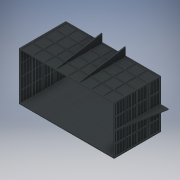
# Autodesk Inventor part: pool cut
Saved by Autodesk Inventor 2019 (Build 230136000, 136)
## iProperties
Created: 2021-05-11
Part Number: pool cut
Material: Stainless Steel, Austenitic
Document SubType Name: Modeling
Designer: jamieson-bl
Density: 8 g/cm^3
Appearance: Semi-Polished
Author: jamieson-bl
Autodesk Inventor part; units mm, degrees
ref_plane "YZ Plane" through (0, 0, 0) normal (1, 0, 0) x (0, 1, 0)
ref_plane "XZ Plane" through (0, 0, 0) normal (0, 1, 0) x (-1, 0, 0)
ref_plane "XY Plane" through (0, 0, 0) normal (0, 0, 1) x (1, 0, 0)
sketch "Sketch1" plane through (0, 0, 0) normal (0, 0, 1) x (1, 0, 0)
  line L0 (1524, -762) -> (-1524, -762)
  line L1 (-1524, -762) -> (-1524, 762)
  line L2 (-1524, 762) -> (1524, 762)
  line L3 (1524, 762) -> (1524, -762)
  line L4 (1524, -762) -> (-1524, 762) construction
  line L5 (-1524, -762) -> (1524, 762) construction
  point P0 (0, 0)
  dimension "d0" = 3048
  dimension "d1" = 1524
  constraints: 12 end point, 2 midpoint, 2 parallel, 1 horizontal, 1 perpendicular
  measures "d0" distance of L1.end L2.end
  measures "d1" distance of L0.end L1.end
extrude "Extrusion1" add sketch "Sketch1" along normal blind 1524
sketch "Sketch2" plane through (0, 0, 1524) normal (0, 0, 1) x (1, 0, 0)
  line L0 (1521.333, -759.333) -> (-1521.333, -759.333)
  line L1 (-1521.333, -759.333) -> (-1521.333, 759.333)
  line L2 (-1521.333, 759.333) -> (1521.333, 759.333)
  line L3 (1521.333, 759.333) -> (1521.333, -759.333)
  line L4 (1521.333, -759.333) -> (-1521.333, 759.333) construction
  line L5 (-1521.333, -759.333) -> (1521.333, 759.333) construction
  point P0 (0, 0)
  dimension "d4" = 3042.666
  dimension "d5" = 1518.666
  constraints: 12 end point, 2 midpoint, 2 parallel, 1 horizontal, 1 perpendicular
  measures "d4" distance of L1.end L2.end
  measures "d5" distance of L0.end L1.end
extrude "Extrusion2" cut sketch "Sketch2" against normal blind 1521.333
sketch "Sketch12" plane through (-1524, 762, 0) normal (0, 1, 0) x (1, 0, 0)
  line L0 (-182.8526, -1524) -> (4734.6574, -1524)
  line L1 (0, -1524) -> (3048, -1524) projected
  line L2 (4734.6574, -1524) -> (4734.6574, -1424)
  line L3 (4734.6574, -1424) -> (-182.8526, -1424)
  line L4 (-182.8526, -1424) -> (-182.8526, -1324)
  line L5 (-182.8526, -1324) -> (4734.6574, -1324)
  line L6 (4734.6574, -1324) -> (4734.6574, -1224)
  line L7 (4734.6574, -1224) -> (-182.8526, -1224)
  line L8 (-182.8526, -1224) -> (-182.8526, -1124)
  line L9 (-182.8526, -1124) -> (4734.6574, -1124)
  line L10 (4734.6574, -1124) -> (4734.6574, -1024)
  line L11 (4734.6574, -1024) -> (-182.8526, -1024)
  line L12 (-182.8526, -1024) -> (-182.8526, -924)
  line L13 (-182.8526, -924) -> (4734.6574, -924)
  line L14 (4734.6574, -924) -> (4734.6574, -824)
  line L15 (4734.6574, -824) -> (-182.8526, -824)
  line L16 (-182.8526, -824) -> (-182.8526, -724)
  line L17 (-182.8526, -724) -> (4734.6574, -724)
  line L18 (4734.6574, -724) -> (4734.6574, -624)
  line L19 (4734.6574, -624) -> (-182.8526, -624)
  line L20 (-182.8526, -624) -> (-182.8526, -524)
  line L21 (-182.8526, -524) -> (4734.6574, -524)
  line L22 (4734.6574, -524) -> (4734.6574, -424)
  line L23 (4734.6574, -424) -> (-182.8526, -424)
  line L24 (-182.8526, -424) -> (-182.8526, -324)
  line L25 (-182.8526, -324) -> (4734.6574, -324)
  line L26 (4734.6574, -324) -> (4734.6574, -224)
  line L27 (4734.6574, -224) -> (-182.8526, -224)
  line L28 (-182.8526, -224) -> (-182.8526, -124)
  line L29 (-182.8526, -124) -> (4734.6574, -124)
  point P0 (1524, 0)
  dimension "d46" = 100
  dimension "d47" = 100
  dimension "d48" = 100
  dimension "d49" = 100
  dimension "d50" = 100
  dimension "d51" = 100
  dimension "d52" = 100
  dimension "d53" = 100
  dimension "d54" = 100
  dimension "d55" = 100
  dimension "d56" = 100
  dimension "d57" = 100
  dimension "d58" = 100
  dimension "d59" = 100
  constraints: 58 end point, 25 point on line, 11 perpendicular, 5 parallel, 1 collinear
  measures "d46" distance of L0.end L2.end
  measures "d47" distance of L3.end L4.end
  measures "d48" distance of L5.end L6.end
  measures "d49" distance of L7.end L8.end
  measures "d50" distance of L9.end L10.end
  measures "d51" distance of L11.end L12.end
  measures "d52" distance of L13.end L14.end
  measures "d53" distance of L15.end L16.end
  measures "d54" distance of L17.end L18.end
  measures "d55" distance of L19.end L20.end
  measures "d56" distance of L21.end L22.end
  measures "d57" distance of L23.end L24.end
  measures "d58" distance of L25.end L26.end
  measures "d59" distance of L27.end L28.end
split_face "Split8"
sketch "Sketch15" plane through (0, 0, 0) normal (0, 0, -1) x (-1, 0, 0)
  line L0 (-1524, 762) -> (-1524, -762) projected
  line L1 (-1524, 762) -> (-1524, 758.825)
  line L2 (-1549.4, 758.825) -> (-1549.4, 787.4)
  line L3 (-1549.4, 787.4) -> (-1498.6, 787.4)
  line L4 (-1498.6, 787.4) -> (-1498.6, 762)
  line L5 (1524, 762) -> (-1524, 762) projected
  line L6 (-1498.6, 762) -> (-1524, 762)
  line L7 (-1549.4, 758.825) -> (-1524, 758.825)
  line L8 (1549.4, -758.825) -> (1524, -758.825)
  line L9 (1549.4, -758.825) -> (1549.4, -787.4)
  line L10 (1549.4, -787.4) -> (1498.6, -787.4)
  line L11 (1498.6, -787.4) -> (1498.6, -762)
  line L12 (1498.6, -762) -> (1524, -762)
  line L13 (1524, -762) -> (1524, -758.825)
  line L14 (0, 0) -> (657.5031, 0) construction
  line L15 (-1524, -762) -> (-1524, 762)
  line L16 (-1524, -762) -> (-1524, -758.825)
  line L17 (-1549.4, -758.825) -> (-1549.4, -787.4)
  line L18 (-1549.4, -787.4) -> (-1498.6, -787.4)
  line L19 (-1498.6, -787.4) -> (-1498.6, -762)
  line L20 (1524, -762) -> (-1524, -762)
  line L21 (-1549.4, -758.825) -> (-1524, -758.825)
  line L22 (1549.4, 758.825) -> (1524, 758.825)
  line L23 (1549.4, 758.825) -> (1549.4, 787.4)
  line L24 (1549.4, 787.4) -> (1498.6, 787.4)
  line L25 (1498.6, 787.4) -> (1498.6, 762)
  line L26 (1498.6, 762) -> (1524, 762)
  line L27 (1524, 762) -> (1524, 758.825)
  line L28 (1524, 762) -> (1524, -762) projected
  line L29 (1524, 762) -> (1549.4, 762)
  line L30 (1549.4, 762) -> (1549.4, 736.6)
  line L31 (1549.4, 736.6) -> (1524, 736.6)
  line L32 (1524, 736.6) -> (1524, 762)
  dimension "d65" = 28.575
  dimension "d68" = 360
  dimension "d134" = 25.4
  dimension "d135" = 25.4
  dimension "d139" = 25.4
  dimension "d141" = 25.4
  constraints: 60 end point, 14 symmetric about line, 3 horizontal, 3 perpendicular, 2 coincident, 2 parallel, 2 point on line, 1 collinear, 1 vertical, 25 other
  measures "d65" distance of L2.start L2.end
  measures "d134" distance of L23.start L22.end
  measures "d135" distance of L25.start L26.start
  measures "d139" distance of L26.end L26.start
  measures "d141" distance of L29.end L30.end
extrude "Extrusion4" add sketch "Sketch15" against normal blind 1524 contours L0 L7 L2 L3 L4 L5 | L0 L20 L19 L18 L17 L21 | L25 L24 L23 L29 L5 | L29 L23 L22 L27 | L12 L13 L8 L9 L10 L11
sketch "Sketch16" plane through (-1498.6, 762, 1524) normal (0, 1, 0) x (1, 0, 0)
  line L0 (0, 1524) -> (2997.2, 1524) projected
  line L1 (0, 1524) -> (0, 0) projected
  line L2 (2997.2, 1524) -> (0, 1524)
  line L3 (0, 1524) -> (0, 1498.6)
  line L4 (0, 1498.6) -> (2997.2, 1498.6)
  line L5 (2997.2, 1498.6) -> (2997.2, 1524)
  line L6 (2997.2, 1123.95) -> (2997.2, 1149.35)
  line L7 (2997.2, 1149.35) -> (0, 1149.35)
  line L8 (0, 1123.95) -> (2997.2, 1123.95)
  line L9 (0, 1149.35) -> (0, 1123.95)
  line L10 (2997.2, 749.3) -> (2997.2, 774.7)
  line L11 (2997.2, 774.7) -> (0, 774.7)
  line L12 (0, 749.3) -> (2997.2, 749.3)
  line L13 (0, 774.7) -> (0, 749.3)
  line L14 (2997.2, 374.65) -> (2997.2, 400.05)
  line L15 (2997.2, 400.05) -> (0, 400.05)
  line L16 (0, 374.65) -> (2997.2, 374.65)
  line L17 (0, 400.05) -> (0, 374.65)
  line L18 (2997.2, 0) -> (2997.2, 25.4)
  line L19 (2997.2, 25.4) -> (0, 25.4)
  line L20 (0, 0) -> (2997.2, 0)
  line L21 (0, 25.4) -> (0, 0)
  point P0 (1498.6, 1524)
  dimension "d72" = 25.4
  dimension "d75" = 374.65
  constraints: 40 end point, 2 parallel, 1 horizontal, 1 perpendicular, 1 point on line, 1 vertical, 32 other
  measures "d72" distance of L3.end L2.end
  measures "d75" distance of L4.end L6.start
extrude "Extrusion5" add sketch "Sketch16" along normal blind 25.4
sketch "Sketch17" plane through (-1498.6, 762, 124) normal (0, 1, 0) x (1, 0, 0)
  line L0 (0, 98.6) -> (2997.2, 98.6) projected
  line L1 (0, -250.65) -> (2997.2, -250.65) projected
  line L2 (1492.123, 98.6) -> (1517.523, 98.6)
  line L3 (1517.523, 98.6) -> (1517.523, -250.65)
  line L4 (1517.523, -250.65) -> (1492.123, -250.65)
  line L5 (1492.123, -250.65) -> (1492.123, 98.6)
  line L6 (1873.123, 98.6) -> (1898.523, 98.6)
  line L7 (1898.523, 98.6) -> (1898.523, -250.65)
  line L8 (1873.123, -250.65) -> (1873.123, 98.6)
  line L9 (1898.523, -250.65) -> (1873.123, -250.65)
  line L10 (2254.123, 98.6) -> (2279.523, 98.6)
  line L11 (2279.523, 98.6) -> (2279.523, -250.65)
  line L12 (2254.123, -250.65) -> (2254.123, 98.6)
  line L13 (2279.523, -250.65) -> (2254.123, -250.65)
  line L14 (2635.123, 98.6) -> (2660.523, 98.6)
  line L15 (2660.523, 98.6) -> (2660.523, -250.65)
  line L16 (2635.123, -250.65) -> (2635.123, 98.6)
  line L17 (2660.523, -250.65) -> (2635.123, -250.65)
  line L18 (1492.123, -276.05) -> (1517.523, -276.05)
  line L19 (1517.523, -276.05) -> (1517.523, -625.3)
  line L20 (1492.123, -625.3) -> (1492.123, -276.05)
  line L21 (1517.523, -625.3) -> (1492.123, -625.3)
  line L22 (1873.123, -276.05) -> (1898.523, -276.05)
  line L23 (1898.523, -276.05) -> (1898.523, -625.3)
  line L24 (1873.123, -625.3) -> (1873.123, -276.05)
  line L25 (1898.523, -625.3) -> (1873.123, -625.3)
  line L26 (2254.123, -276.05) -> (2279.523, -276.05)
  line L27 (2279.523, -276.05) -> (2279.523, -625.3)
  line L28 (2254.123, -625.3) -> (2254.123, -276.05)
  line L29 (2279.523, -625.3) -> (2254.123, -625.3)
  line L30 (2635.123, -276.05) -> (2660.523, -276.05)
  line L31 (2660.523, -276.05) -> (2660.523, -625.3)
  line L32 (2635.123, -625.3) -> (2635.123, -276.05)
  line L33 (2660.523, -625.3) -> (2635.123, -625.3)
  line L34 (1492.123, -650.7) -> (1517.523, -650.7)
  line L35 (1517.523, -650.7) -> (1517.523, -999.95)
  line L36 (1492.123, -999.95) -> (1492.123, -650.7)
  line L37 (1517.523, -999.95) -> (1492.123, -999.95)
  line L38 (1873.123, -650.7) -> (1898.523, -650.7)
  line L39 (1898.523, -650.7) -> (1898.523, -999.95)
  line L40 (1873.123, -999.95) -> (1873.123, -650.7)
  line L41 (1898.523, -999.95) -> (1873.123, -999.95)
  line L42 (2254.123, -650.7) -> (2279.523, -650.7)
  line L43 (2279.523, -650.7) -> (2279.523, -999.95)
  line L44 (2254.123, -999.95) -> (2254.123, -650.7)
  line L45 (2279.523, -999.95) -> (2254.123, -999.95)
  line L46 (2635.123, -650.7) -> (2660.523, -650.7)
  line L47 (2660.523, -650.7) -> (2660.523, -999.95)
  line L48 (2635.123, -999.95) -> (2635.123, -650.7)
  line L49 (2660.523, -999.95) -> (2635.123, -999.95)
  line L50 (1492.123, -1025.35) -> (1517.523, -1025.35)
  line L51 (1517.523, -1025.35) -> (1517.523, -1374.6)
  line L52 (1492.123, -1374.6) -> (1492.123, -1025.35)
  line L53 (1517.523, -1374.6) -> (1492.123, -1374.6)
  line L54 (1873.123, -1025.35) -> (1898.523, -1025.35)
  line L55 (1898.523, -1025.35) -> (1898.523, -1374.6)
  line L56 (1873.123, -1374.6) -> (1873.123, -1025.35)
  line L57 (1898.523, -1374.6) -> (1873.123, -1374.6)
  line L58 (2254.123, -1025.35) -> (2279.523, -1025.35)
  line L59 (2279.523, -1025.35) -> (2279.523, -1374.6)
  line L60 (2254.123, -1374.6) -> (2254.123, -1025.35)
  line L61 (2279.523, -1374.6) -> (2254.123, -1374.6)
  line L62 (2635.123, -1025.35) -> (2660.523, -1025.35)
  line L63 (2660.523, -1025.35) -> (2660.523, -1374.6)
  line L64 (2635.123, -1374.6) -> (2635.123, -1025.35)
  line L65 (2660.523, -1374.6) -> (2635.123, -1374.6)
  line L66 (1136.523, 98.6) -> (1136.523, -250.65)
  line L67 (1111.123, 98.6) -> (1136.523, 98.6)
  line L68 (1111.123, -250.65) -> (1111.123, 98.6)
  line L69 (1136.523, -250.65) -> (1111.123, -250.65)
  line L70 (1111.123, -276.05) -> (1136.523, -276.05)
  line L71 (1136.523, -276.05) -> (1136.523, -625.3)
  line L72 (1111.123, -625.3) -> (1111.123, -276.05)
  line L73 (1136.523, -625.3) -> (1111.123, -625.3)
  line L74 (1111.123, -650.7) -> (1136.523, -650.7)
  line L75 (1136.523, -650.7) -> (1136.523, -999.95)
  line L76 (1111.123, -999.95) -> (1111.123, -650.7)
  line L77 (1136.523, -999.95) -> (1111.123, -999.95)
  line L78 (1111.123, -1025.35) -> (1136.523, -1025.35)
  line L79 (1136.523, -1025.35) -> (1136.523, -1374.6)
  line L80 (1111.123, -1374.6) -> (1111.123, -1025.35)
  line L81 (1136.523, -1374.6) -> (1111.123, -1374.6)
  line L82 (755.523, 98.6) -> (755.523, -250.65)
  line L83 (730.123, 98.6) -> (755.523, 98.6)
  line L84 (730.123, -250.65) -> (730.123, 98.6)
  line L85 (755.523, -250.65) -> (730.123, -250.65)
  line L86 (730.123, -276.05) -> (755.523, -276.05)
  line L87 (755.523, -276.05) -> (755.523, -625.3)
  line L88 (730.123, -625.3) -> (730.123, -276.05)
  line L89 (755.523, -625.3) -> (730.123, -625.3)
  line L90 (730.123, -650.7) -> (755.523, -650.7)
  line L91 (755.523, -650.7) -> (755.523, -999.95)
  line L92 (730.123, -999.95) -> (730.123, -650.7)
  line L93 (755.523, -999.95) -> (730.123, -999.95)
  line L94 (730.123, -1025.35) -> (755.523, -1025.35)
  line L95 (755.523, -1025.35) -> (755.523, -1374.6)
  line L96 (730.123, -1374.6) -> (730.123, -1025.35)
  line L97 (755.523, -1374.6) -> (730.123, -1374.6)
  line L98 (374.523, 98.6) -> (374.523, -250.65)
  line L99 (349.123, 98.6) -> (374.523, 98.6)
  line L100 (349.123, -250.65) -> (349.123, 98.6)
  line L101 (374.523, -250.65) -> (349.123, -250.65)
  line L102 (349.123, -276.05) -> (374.523, -276.05)
  line L103 (374.523, -276.05) -> (374.523, -625.3)
  line L104 (349.123, -625.3) -> (349.123, -276.05)
  line L105 (374.523, -625.3) -> (349.123, -625.3)
  line L106 (349.123, -650.7) -> (374.523, -650.7)
  line L107 (374.523, -650.7) -> (374.523, -999.95)
  line L108 (349.123, -999.95) -> (349.123, -650.7)
  line L109 (374.523, -999.95) -> (349.123, -999.95)
  line L110 (349.123, -1025.35) -> (374.523, -1025.35)
  line L111 (374.523, -1025.35) -> (374.523, -1374.6)
  line L112 (349.123, -1374.6) -> (349.123, -1025.35)
  line L113 (374.523, -1374.6) -> (349.123, -1374.6)
  point P0 (1498.6, 124)
  dimension "d82" = 25.4
  dimension "d85" = 381
  dimension "d88" = 374.65
  dimension "d93" = 381
  constraints: 224 end point, 3 horizontal, 2 parallel, 2 point on line, 1 collinear, 1 perpendicular, 1 vertical, 215 other
  measures "d82" distance of L3.end L4.end
  measures "d85" distance of L2.start L6.start
  measures "d88" distance of L2.start L18.start
  measures "d93" distance of L2.end L66.start
extrude "Extrusion6" add sketch "Sketch17" along normal blind 25.4 contours L0 L98 L1 L100 | L0 L82 L1 L84 | L0 L66 L1 L68 | L0 L3 L1 L5 | L0 L7 L1 L8 | L0 L11 L1 L12 | L0 L15 L1 L16 | L18 L19 L21 L20 | L22 L23 L25 L24 | L26 L27 L29 L28 | L30 L31 L33 L32 | L34 L35 L37 L36 | L38 L39 L41 L40 | L42 L43 L45 L44 | L46 L47 L49 L48 | L50 L51 L53 L52 | L54 L55 L57 L56 | L58 L59 L61 L60 | L62 L63 L65 L64 | L70 L71 L73 L72 | L74 L75 L77 L76 | L78 L79 L81 L80 | L86 L87 L89 L88 | L90 L91 L93 L92 | L94 L95 L97 L96 | L102 L103 L105 L104 | L106 L107 L109 L108 | L110 L111 L113 L112
pattern_linear "Rectangular Pattern1" count 2 spacing 1549.4 along (0, -1, 0) of "Extrusion6", "Extrusion5"
sketch "Sketch18" plane through (1524, -758.825, 524) normal (1, 0, 0) x (0, 0, -1)
  line L0 (524, 1517.65) -> (-1000, 1517.65) projected
  line L1 (524, 0) -> (-1000, 0) projected
  line L2 (-1000, 1517.65) -> (-974.6, 1517.65)
  line L3 (-974.6, 1517.65) -> (-974.6, 0)
  line L4 (-974.6, 0) -> (-1000, 0)
  line L5 (-1000, 0) -> (-1000, 1517.65)
  line L6 (-599.95, 1517.65) -> (-599.95, 0)
  line L7 (-625.35, 1517.65) -> (-599.95, 1517.65)
  line L8 (-625.35, 0) -> (-625.35, 1517.65)
  line L9 (-599.95, 0) -> (-625.35, 0)
  line L10 (-225.3, 1517.65) -> (-225.3, 0)
  line L11 (-250.7, 1517.65) -> (-225.3, 1517.65)
  line L12 (-250.7, 0) -> (-250.7, 1517.65)
  line L13 (-225.3, 0) -> (-250.7, 0)
  line L14 (149.35, 1517.65) -> (149.35, 0)
  line L15 (123.95, 1517.65) -> (149.35, 1517.65)
  line L16 (123.95, 0) -> (123.95, 1517.65)
  line L17 (149.35, 0) -> (123.95, 0)
  line L18 (524, 1517.65) -> (524, 0)
  line L19 (498.6, 1517.65) -> (524, 1517.65)
  line L20 (498.6, 0) -> (498.6, 1517.65)
  line L21 (524, 0) -> (498.6, 0)
  point P0 (524, 758.825)
  dimension "d103" = 25.4
  dimension "d106" = 374.65
  constraints: 40 end point, 2 horizontal, 2 parallel, 1 perpendicular, 1 point on line, 32 other
  measures "d103" distance of L3.end L4.end
  measures "d106" distance of L2.end L6.start
extrude "Extrusion7" add sketch "Sketch18" along normal blind 25.4 contours L18 L1 L20 L0 | L14 L1 L16 L0 | L10 L1 L12 L0 | L6 L1 L8 L0 | L3 L1 L5 L0
sketch "Sketch19" plane through (1524, -758.825, 1424) normal (1, 0, 0) x (0, 0, -1)
  line L0 (1398.6, 1517.65) -> (1398.6, 0) projected
  line L1 (1049.35, 0) -> (1049.35, 1517.65) projected
  line L2 (1398.6, 723.9) -> (1049.35, 723.9)
  line L3 (1049.35, 723.9) -> (1049.35, 749.3)
  line L4 (1049.35, 749.3) -> (1398.6, 749.3)
  line L5 (1398.6, 749.3) -> (1398.6, 723.9)
  line L6 (1049.35, 1104.9) -> (1049.35, 1130.3)
  line L7 (1049.35, 1130.3) -> (1398.6, 1130.3)
  line L8 (1398.6, 1104.9) -> (1049.35, 1104.9)
  line L9 (1398.6, 1130.3) -> (1398.6, 1104.9)
  line L10 (674.7, 723.9) -> (674.7, 749.3)
  line L11 (674.7, 749.3) -> (1023.95, 749.3)
  line L12 (1023.95, 723.9) -> (674.7, 723.9)
  line L13 (1023.95, 749.3) -> (1023.95, 723.9)
  line L14 (674.7, 1104.9) -> (674.7, 1130.3)
  line L15 (674.7, 1130.3) -> (1023.95, 1130.3)
  line L16 (1023.95, 1104.9) -> (674.7, 1104.9)
  line L17 (1023.95, 1130.3) -> (1023.95, 1104.9)
  line L18 (300.05, 723.9) -> (300.05, 749.3)
  line L19 (300.05, 749.3) -> (649.3, 749.3)
  line L20 (649.3, 723.9) -> (300.05, 723.9)
  line L21 (649.3, 749.3) -> (649.3, 723.9)
  line L22 (300.05, 1104.9) -> (300.05, 1130.3)
  line L23 (300.05, 1130.3) -> (649.3, 1130.3)
  line L24 (649.3, 1104.9) -> (300.05, 1104.9)
  line L25 (649.3, 1130.3) -> (649.3, 1104.9)
  line L26 (-74.6, 723.9) -> (-74.6, 749.3)
  line L27 (-74.6, 749.3) -> (274.65, 749.3)
  line L28 (274.65, 723.9) -> (-74.6, 723.9)
  line L29 (274.65, 749.3) -> (274.65, 723.9)
  line L30 (-74.6, 1104.9) -> (-74.6, 1130.3)
  line L31 (-74.6, 1130.3) -> (274.65, 1130.3)
  line L32 (274.65, 1104.9) -> (-74.6, 1104.9)
  line L33 (274.65, 1130.3) -> (274.65, 1104.9)
  line L34 (1049.35, 368.3) -> (1398.6, 368.3)
  line L35 (1398.6, 342.9) -> (1049.35, 342.9)
  line L36 (1398.6, 368.3) -> (1398.6, 342.9)
  line L37 (1049.35, 342.9) -> (1049.35, 368.3)
  line L38 (1023.95, 368.3) -> (1023.95, 342.9)
  line L39 (674.7, 368.3) -> (1023.95, 368.3)
  line L40 (1023.95, 342.9) -> (674.7, 342.9)
  line L41 (674.7, 342.9) -> (674.7, 368.3)
  line L42 (649.3, 368.3) -> (649.3, 342.9)
  line L43 (300.05, 368.3) -> (649.3, 368.3)
  line L44 (649.3, 342.9) -> (300.05, 342.9)
  line L45 (300.05, 342.9) -> (300.05, 368.3)
  line L46 (274.65, 368.3) -> (274.65, 342.9)
  line L47 (-74.6, 368.3) -> (274.65, 368.3)
  line L48 (274.65, 342.9) -> (-74.6, 342.9)
  line L49 (-74.6, 342.9) -> (-74.6, 368.3)
  point P0 (1424, 758.825)
  dimension "d113" = 25.4
  dimension "d116" = 381
  dimension "d119" = 374.65
  dimension "d124" = 381
  constraints: 96 end point, 2 horizontal, 2 parallel, 2 point on line, 2 vertical, 1 collinear, 1 perpendicular, 87 other
  measures "d113" distance of L2.end L3.end
  measures "d116" distance of L2.end L6.start
  measures "d119" distance of L2.end L10.start
  measures "d124" distance of L3.end L34.start
extrude "Extrusion8" add sketch "Sketch19" along normal blind 25.4 contours L0 L8 L1 L7 | L0 L2 L1 L4 | L0 L35 L1 L34 | L10 L11 L13 L12 | L14 L15 L17 L16 | L18 L19 L21 L20 | L22 L23 L25 L24 | L26 L27 L29 L28 | L30 L31 L33 L32 | L38 L40 L41 L39 | L42 L44 L45 L43 | L46 L48 L49 L47
pattern_linear "Rectangular Pattern3" count 2 spacing 3073.4 along (-1, 0, 0) of "Extrusion7", "Extrusion8"
sketch "Sketch20" plane through (-387.477, -787.4, 1149.35) normal (-1, 0, 0) x (0, 0, 1)
  line L0 (374.65, 0) -> (374.65, 1574.8) projected
  line L1 (374.65, 0) -> (-1149.35, 0)
  line L2 (-1149.35, 0) -> (-1149.35, -254)
  line L3 (-1149.35, -254) -> (374.65, 0)
  point P0 (-1149.35, 787.4)
  dimension "d142" = 254
  constraints: 6 end point, 1 horizontal, 1 perpendicular
  measures "d142" distance of L1.end L2.end
extrude "Extrusion9" add sketch "Sketch20" against normal blind 25.4
pattern_linear "Rectangular Pattern4" count 2 spacing 762 along (1, 0, 0) of "Extrusion9"
mirror "Mirror1" about plane through (0, 0, 0) normal (0, 1, 0) of "Extrusion9", "Rectangular Pattern4"
sketch "Sketch21" plane through (1524, -34.925, 1324) normal (0, -1, 0) x (1, 0, 0)
  line L0 (-1124.077, 200) -> (25.4, 200) projected
  line L1 (25.4, 200) -> (25.4, -1324)
  line L2 (25.4, -1324) -> (279.4, -1324)
  line L3 (279.4, -1324) -> (25.4, 200)
  point P0 (-1524, -1324)
  point P1 (-25.4, 200)
  dimension "d148" = 254
  constraints: 6 end point, 1 perpendicular, 1 vertical
  measures "d148" distance of L1.end L2.end
extrude "Extrusion10" add sketch "Sketch21" against normal blind 25.4
mirror "Mirror2" about plane through (0, 0, 0) normal (1, 0, 0) of "Extrusion10"
